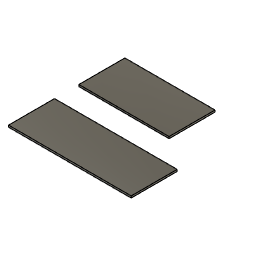
tray-divider (Autodesk Fusion 360 design; units mm, degrees)
Autodesk Fusion 360 part; units mm, degrees
sketch "Sketch1" plane through (0, 0, 0) normal (0, 0, 1) x (1, 0, 0)
  line L0 (0, 0) -> (50, 0)
  line L1 (50, 0) -> (50, 25.5)
  line L2 (50, 25.5) -> (0, 25.5)
  line L3 (0, 25.5) -> (0, 0)
  dimension "d1" = 50
  dimension "d2" = 25.5
  constraint horizontal L0
  constraint vertical L1
  constraint horizontal L2
  constraint vertical L3
  constraint coincident L0.start L3.end
  measures "d1" distance of L0.start L0.end
  measures "d2" distance of L0.start L2.end
extrude "Extrude1" add sketch "Sketch1" along normal blind 1 makes body 1
copy_body "CopyPasteBodies1" bodies 1 makes body 2
move_body "Move1" bodies 2 to x (1, 0, 0) y (0, 1, 0) z (0, 0, 1) at (0, -39, 0)
move_face "OffsetFaces1" offset 18 1 faces at (50, -30.5, 0.3333) on bodies 2
named bodies: "tray-divider", "tray-divider-long"
